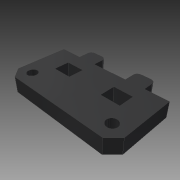
# Autodesk Inventor part: y_carriage_belt_mount
Saved by Autodesk Inventor 2014 (Build 180170000, 170)
## iProperties
Created: 2013-11-29
Part Number: y_carriage_belt_mount
Material: Plywood, Finish
Document SubType Name: Modeling
Designer: buben
Density: 0.552 g/cm^3
Appearance: Plywood - New
Author: buben
Subject: Laser Cutted
Autodesk Inventor part; units mm, degrees
ref_plane "YZ Plane" through (0, 0, 0) normal (1, 0, 0) x (0, 1, 0)
ref_plane "XZ Plane" through (0, 0, 0) normal (0, 1, 0) x (-1, 0, 0)
ref_plane "XY Plane" through (0, 0, 0) normal (0, 0, 1) x (1, 0, 0)
sketch "Sketch1" plane through (0, 0, 0) normal (0, 0, 1) x (1, 0, 0)
  line L0 (4, 0) -> (46, 0)
  line L1 (50, 4) -> (50, 26)
  line L2 (50, 26) -> (0, 26)
  line L3 (0, 26) -> (0, 4)
  line L4 (0, 4) -> (4, 0)
  line L5 (46, 0) -> (50, 4)
  circle A0 centre (6, 6) radius 2.25
  circle A1 centre (44, 6) radius 2.25
  line L6 (9.5, 20) -> (17.5, 20)
  line L7 (17.5, 20) -> (17.5, 13.5)
  line L8 (17.5, 13.5) -> (9.5, 13.5)
  line L9 (9.5, 13.5) -> (9.5, 20)
  line L10 (32.5, 20) -> (40.5, 20)
  line L11 (40.5, 20) -> (40.5, 13.5)
  line L12 (40.5, 13.5) -> (32.5, 13.5)
  line L13 (32.5, 13.5) -> (32.5, 20)
  line L14 (17.5, 20) -> (32.5, 13.5) construction
  line L15 (32.5, 20) -> (17.5, 13.5) construction
  point P0 (0, 0)
  point P1 (50, 0)
  point P2 (25, 16.75)
  point P3 (25, 26)
  dimension "d0" = 26
  dimension "d1" = 50
  dimension "d2" = 4
  dimension "d3" = 4
  dimension "d4" = 4
  dimension "d5" = 4
  dimension "d6" = 4.5
  dimension "d7" = 4.5
  dimension "d8" = 20
  dimension "d9" = 6
  dimension "d10" = 6
  dimension "d11" = 6.5
  dimension "d12" = 8
  dimension "d13" = 8
  dimension "d14" = 15
  dimension "d15" = 6
  constraints: 32 end point, 6 parallel, 4 point on line, 3 horizontal, 3 perpendicular, 2 centre point, 2 collinear, 2 midpoint, 1 horizontal alignment, 1 vertical alignment
  measures "d0" distance of L2.end point (0, 0)
  measures "d1" distance of point (0, 0) point (50, 0)
  measures "d2" distance of L3.end point (0, 0)
  measures "d3" distance of L0.start point (0, 0)
  measures "d4" distance of L0.end point (50, 0)
  measures "d5" distance of L1.start point (50, 0)
  measures "d6" diameter of A1
  measures "d7" diameter of A0
  measures "d8" distance from line of L2 A0.centre
  measures "d9" distance from line of L3 A0.centre
  measures "d10" distance from line of L1 A1.centre
  measures "d11" distance of L8.end L6.start
  measures "d12" distance of L6.start L6.end
  measures "d13" distance of L10.start L10.end
  measures "d14" distance between parallel lines of L13 L7
  measures "d15" distance between parallel lines of L2 L6
extrude "Extrusion1" add sketch "Sketch1" along normal blind 6.5
sketch "Sketch2" plane through (0, 0, 6.5) normal (0, 0, 1) x (1, 0, 0)
  line L0 (17.5, 20) -> (17.5, 13.5) projected
  line L1 (50, 26) -> (0, 26) projected
  line L2 (9.5, 26) -> (17.5, 26)
  line L3 (17.5, 26) -> (17.5, 30.5)
  line L4 (15.5, 32.5) -> (11.5, 32.5)
  line L5 (9.5, 30.5) -> (9.5, 26)
  line L6 (32.5, 26) -> (40.5, 26)
  line L7 (40.5, 26) -> (40.5, 30.5)
  line L8 (38.5, 32.5) -> (34.5, 32.5)
  line L9 (32.5, 30.5) -> (32.5, 26)
  arc A0 (11.5, 32.5) -> (9.5, 30.5) centre (11.5, 30.5) ccw
  arc A1 (17.5, 30.5) -> (15.5, 32.5) centre (15.5, 30.5) ccw
  arc A2 (34.5, 32.5) -> (32.5, 30.5) centre (34.5, 30.5) ccw
  arc A3 (40.5, 30.5) -> (38.5, 32.5) centre (38.5, 30.5) ccw
  point P0 (0, 0)
  dimension "d18" = 2
  dimension "d19" = 8
  dimension "d20" = 8
  dimension "d21" = 15
  dimension "d22" = 6.5
  constraints: 16 end point, 8 point on circle, 8 tangent, 4 centre point, 4 parallel, 3 equal radius, 2 collinear, 2 horizontal, 2 perpendicular, 2 point on line
  measures "d18" radius of A0
  measures "d19" distance between parallel lines of L3 L5
  measures "d20" distance between parallel lines of L7 L9
  measures "d21" distance between parallel lines of L9 L3
  measures "d22" distance between parallel lines of L2 L4
extrude "Extrusion2" add sketch "Sketch2" against normal blind 6.5
equation "\"d3\" = d2"
equation "\"d4\" = d2"
equation "\"d5\" = d4"
body "Solid1"
